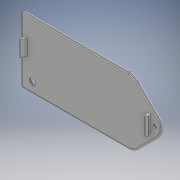
# Autodesk Inventor part: Arduino simple 4 channel ttl top
Saved by Autodesk Inventor 2017 (Build 210142000, 142)
## iProperties
Created: 2016-10-04
Part Number: Arduino simple 4 channel ttl top
Material: Generic
Document SubType Name: Modeling
Designer: andrew
Density: 1 g/cm^3
Appearance: Default
Author: andrew
Autodesk Inventor part; units mm, degrees
ref_plane "YZ Plane" through (0, 0, 0) normal (1, 0, 0) x (0, 1, 0)
ref_plane "XZ Plane" through (0, 0, 0) normal (0, 1, 0) x (-1, 0, 0)
ref_plane "XY Plane" through (0, 0, 0) normal (0, 0, 1) x (1, 0, 0)
sketch "Sketch1" plane through (0, 0, 0) normal (0, 1, 0) x (-1, 0, 0)
  line L0 (70.1002, -51.1999) -> (70.1002, -37.9894) construction
  line L1 (70.1002, -37.9894) -> (68.1002, -37.9894) construction
  line L2 (68.1002, -37.9894) -> (68.1002, -48.1999) construction
  arc A0 (67.1002, -49.1999) -> (68.1002, -48.1999) centre (67.1002, -48.1999) ccw construction
  line L3 (67.1002, -49.1999) -> (-5.9213, -49.1999) construction
  arc A1 (-7.3356, -48.6141) -> (-5.9213, -49.1999) centre (-5.9213, -47.1999) ccw construction
  line L4 (-7.3356, -48.6141) -> (-7.664, -48.2857) construction
  arc A2 (-7.664, -48.2857) -> (-9.0782, -47.6999) centre (-9.0782, -49.6999) ccw construction
  line L5 (-9.0782, -47.6999) -> (-35.9958, -47.6999) construction
  arc A3 (-42.0062, -45.2103) -> (-35.9958, -47.6999) centre (-35.9958, -39.1999) ccw construction
  line L6 (-42.0062, -45.2103) -> (-62.1562, -25.0603) construction
  arc A4 (-62.1562, -13.0395) -> (-62.1562, -25.0603) centre (-56.1458, -19.0499) ccw construction
  line L7 (-62.1562, -13.0395) -> (-42.0062, 7.1105) construction
  arc A5 (-35.9958, 9.6001) -> (-42.0062, 7.1105) centre (-35.9958, 1.1001) ccw construction
  line L8 (-35.9958, 9.6001) -> (-9.0782, 9.6001) construction
  arc A6 (-9.0782, 9.6001) -> (-7.664, 10.1859) centre (-9.0782, 11.6001) ccw construction
  line L9 (-7.664, 10.1859) -> (-7.3356, 10.5143) construction
  arc A7 (-5.9213, 11.1001) -> (-7.3356, 10.5143) centre (-5.9213, 9.1001) ccw construction
  line L10 (-5.9213, 11.1001) -> (67.1002, 11.1001) construction
  arc A8 (68.1002, 10.1001) -> (67.1002, 11.1001) centre (67.1002, 10.1001) ccw construction
  line L11 (68.1002, 10.1001) -> (68.1002, 5.7045) construction
  line L12 (68.1002, 5.7045) -> (70.1002, 5.7045) construction
  line L13 (70.1002, 5.7045) -> (70.1002, 13.1001) construction
  line L14 (70.1002, 13.1001) -> (-35.9958, 13.1001) construction
  arc A9 (-35.9958, 13.1001) -> (-44.4811, 9.5854) centre (-35.9958, 1.1001) ccw construction
  line L15 (-44.4811, 9.5854) -> (-64.6311, -10.5646) construction
  arc A10 (-64.6311, -10.5646) -> (-64.6311, -27.5352) centre (-56.1458, -19.0499) ccw construction
  line L16 (-64.6311, -27.5352) -> (-44.4811, -47.6852) construction
  arc A11 (-44.4811, -47.6852) -> (-35.9958, -51.1999) centre (-35.9958, -39.1999) ccw construction
  line L17 (-35.9958, -51.1999) -> (70.1002, -51.1999) construction
  line L18 (70.1002, -21.9894) -> (70.1002, -6.0043) construction
  line L19 (70.1002, -6.0043) -> (68.1002, -6.0043) construction
  line L20 (68.1002, -6.0043) -> (68.1002, -21.9894) construction
  line L21 (68.1002, -21.9894) -> (70.1002, -21.9894) construction
  line L22 (71.1002, -21.9894) -> (71.1002, -6.0043) construction
  line L23 (71.1002, 5.7045) -> (71.1002, 13.1001)
  arc A12 (71.1002, 13.1001) -> (70.1002, 14.1001) centre (70.1002, 13.1001) ccw
  line L24 (70.1002, 14.1001) -> (-35.9958, 14.1001)
  arc A13 (-35.9958, 14.1001) -> (-45.1882, 10.2925) centre (-35.9958, 1.1001) ccw
  line L25 (-45.1882, 10.2925) -> (-65.3382, -9.8575)
  arc A14 (-65.3382, -9.8575) -> (-65.3382, -28.2423) centre (-56.1458, -19.0499) ccw
  line L26 (-65.3382, -28.2423) -> (-45.1882, -48.3923)
  arc A15 (-45.1882, -48.3923) -> (-35.9958, -52.1999) centre (-35.9958, -39.1999) ccw
  line L27 (-35.9958, -52.1999) -> (70.1002, -52.1999)
  arc A16 (70.1002, -52.1999) -> (71.1002, -51.1999) centre (70.1002, -51.1999) ccw
  line L28 (71.1002, -51.1999) -> (71.1002, -37.9894)
  line L29 (71.1002, -37.9894) -> (70.1002, -37.9894) construction
  line L30 (70.1002, -37.9894) -> (70.1002, -51.1999) construction
  line L31 (70.1002, -51.1999) -> (-35.9958, -51.1999) construction
  arc A17 (-44.4811, -47.6852) -> (-35.9958, -51.1999) centre (-35.9958, -39.1999) ccw construction
  line L32 (-44.4811, -47.6852) -> (-64.6311, -27.5352) construction
  arc A18 (-64.6311, -10.5646) -> (-64.6311, -27.5352) centre (-56.1458, -19.0499) ccw construction
  line L33 (-64.6311, -10.5646) -> (-44.4811, 9.5854) construction
  arc A19 (-35.9958, 13.1001) -> (-44.4811, 9.5854) centre (-35.9958, 1.1001) ccw construction
  line L34 (-35.9958, 13.1001) -> (70.1002, 13.1001) construction
  line L35 (70.1002, 13.1001) -> (70.1002, 5.7045) construction
  line L36 (70.1002, 5.7045) -> (71.1002, 5.7045) construction
  line L37 (71.1002, 5.7045) -> (71.1002, 13.1001)
  line L38 (71.1002, 5.7045) -> (71.1002, -37.9894)
  arc A20 (-62.1562, -13.0395) -> (-62.1562, -25.0603) centre (-56.1458, -19.0499) ccw construction
  line L39 (-64.6458, -19.0499) -> (-76.6779, -19.0499) construction
  arc A21 (-65.3382, -9.8575) -> (-65.3382, -28.2423) centre (-56.1458, -19.0499) ccw
  circle A22 centre (-63.0458, -19.0499) radius 1.8
  point P0 (0, 0)
  point P1 (66.1, 7.6)
  point P2 (-59.329, -19.0499)
  constraints: 80 end point, 45 point on circle, 23 centre point, 1 vertical
extrude "Extrusion1" add sketch "Sketch1" along normal blind 3
sketch "Sketch2" plane through (0, 0, 0) normal (0, -1, 0) x (1, 0, 0)
  arc A0 (-71.1002, -51.1999) -> (-70.1002, -52.1999) centre (-70.1002, -51.1999) ccw projected
  line L0 (-71.1002, 13.1001) -> (-71.1002, -0.1104)
  line L1 (-70.1002, -0.1104) -> (-68.1002, -0.1104) construction
  line L2 (-68.1002, -0.1104) -> (-68.1002, 10.1001) construction
  arc A1 (-67.1002, 11.1001) -> (-68.1002, 10.1001) centre (-67.1002, 10.1001) ccw construction
  line L3 (-68.1002, -16.1104) -> (-70.1002, -16.1104) construction
  line L4 (-70.1002, -16.1104) -> (-70.1002, -32.0955) construction
  line L5 (-71.1002, -16.1104) -> (-71.1002, -32.0955) construction
  line L6 (-70.1002, -32.0955) -> (-68.1002, -32.0955) construction
  line L7 (-68.1002, -32.0955) -> (-68.1002, -16.1104) construction
  line L8 (-71.1002, -43.8043) -> (-71.1002, -0.1104)
  line L9 (-67.1002, 11.1001) -> (5.9213, 11.1001) construction
  line L10 (35.9958, 14.1001) -> (-70.1002, 14.1001)
  line L11 (35.9958, 13.1001) -> (-70.1002, 13.1001) construction
  line L12 (5.9213, -49.1999) -> (-67.1002, -49.1999) construction
  line L13 (-70.1002, -51.1999) -> (35.9958, -51.1999) construction
  line L14 (-70.1002, -52.1999) -> (35.9958, -52.1999)
  line L15 (-70.1002, 13.1001) -> (-70.1002, -0.1104) construction
  arc A2 (-70.1002, 14.1001) -> (-71.1002, 13.1001) centre (-70.1002, 13.1001) ccw
  line L16 (-68.1002, -43.8043) -> (-70.1002, -43.8043) construction
  line L17 (-68.1002, -48.1999) -> (-68.1002, -43.8043) construction
  arc A3 (-68.1002, -48.1999) -> (-67.1002, -49.1999) centre (-67.1002, -48.1999) ccw construction
  line L18 (-71.1002, -43.8043) -> (-71.1002, -51.1999)
  line L19 (-71.1002, -43.8043) -> (-71.1002, -51.1999)
  line L20 (-70.1002, -43.8043) -> (-70.1002, -51.1999) construction
  arc A4 (-71.1002, -51.1999) -> (-70.1002, -52.1999) centre (-70.1002, -51.1999) ccw
  arc A5 (5.9213, -49.1999) -> (7.3356, -48.6141) centre (5.9213, -47.1999) ccw construction
  arc A6 (9.0782, -47.6999) -> (7.664, -48.2857) centre (9.0782, -49.6999) ccw construction
  line L21 (35.9958, -47.6999) -> (9.0782, -47.6999) construction
  arc A7 (35.9958, -47.6999) -> (42.0062, -45.2103) centre (35.9958, -39.1999) ccw construction
  arc A8 (35.9958, -52.1999) -> (45.1882, -48.3923) centre (35.9958, -39.1999) ccw
  line L22 (7.664, -48.2857) -> (7.3356, -48.6141) construction
  line L23 (62.1562, -25.0603) -> (42.0062, -45.2103) construction
  line L24 (45.1882, -48.3923) -> (65.3382, -28.2423)
  arc A9 (62.1562, -25.0603) -> (62.1562, -13.0395) centre (56.1458, -19.0499) ccw construction
  arc A10 (65.3382, -28.2423) -> (65.3382, -9.8575) centre (56.1458, -19.0499) ccw
  arc A11 (7.3356, 10.5143) -> (5.9213, 11.1001) centre (5.9213, 9.1001) ccw construction
  arc A12 (7.664, 10.1859) -> (9.0782, 9.6001) centre (9.0782, 11.6001) ccw construction
  line L25 (9.0782, 9.6001) -> (35.9958, 9.6001) construction
  line L26 (7.3356, 10.5143) -> (7.664, 10.1859) construction
  line L27 (42.0062, 7.1105) -> (62.1562, -13.0395) construction
  line L28 (65.3382, -9.8575) -> (45.1882, 10.2925)
  arc A13 (42.0062, 7.1105) -> (35.9958, 9.6001) centre (35.9958, 1.1001) ccw construction
  arc A14 (44.4811, 9.5854) -> (35.9958, 13.1001) centre (35.9958, 1.1001) ccw construction
  arc A15 (45.1882, 10.2925) -> (35.9958, 14.1001) centre (35.9958, 1.1001) ccw
  line L29 (-69.6002, 12.6001) -> (35.9958, 12.6001)
  arc A16 (44.1275, 9.2318) -> (35.9958, 12.6001) centre (35.9958, 1.1001) ccw
  line L30 (44.1275, 9.2318) -> (64.2775, -10.9182)
  arc A17 (64.2775, -27.1816) -> (64.2775, -10.9182) centre (56.1458, -19.0499) ccw
  line L31 (64.2775, -27.1816) -> (44.1275, -47.3316)
  arc A18 (35.9958, -50.6999) -> (44.1275, -47.3316) centre (35.9958, -39.1999) ccw
  line L32 (35.9958, -50.6999) -> (-69.6002, -50.6999)
  line L33 (-69.6002, -50.6999) -> (-69.6002, 12.6001)
  point P0 (0, -38.0998)
  point P1 (-66.1, -45.6998)
  constraints: 68 end point, 36 point on circle, 18 centre point, 1 vertical
extrude "Extrusion2" cut sketch "Sketch2" against normal blind 1
fillet "Fillet1" radius 2 10 edges at (40.9707, 3, 13.1105) (55.2632, 3, 0.2175) (69.1458, 3, -19.0499) (55.2632, 3, -38.3173) (40.9707, 3, -51.2103) (-17.0522, 3, -52.1999) (-70.8073, 3, -51.907) (-71.1002, 3, -19.0499) (-70.8073, 3, 13.8072) (-17.0522, 3, 14.1001)
sketch "Sketch3" plane through (0, 0, 0) normal (0, -1, 0) x (1, 0, 0)
  arc A0 (65.3382, -28.2423) -> (65.3382, -9.8575) centre (56.1458, -19.0499) ccw construction
  line L0 (-70.1002, -43.8043) -> (-71.1002, -43.8043) construction
  line L1 (-70.1002, -43.8043) -> (-70.1002, -51.1999) construction
  line L2 (-70.1002, -51.1999) -> (-70.1002, -43.8043) construction
  line L3 (-68.1002, -48.1999) -> (-68.1002, -43.8043) construction
  line L4 (-68.1002, -43.8043) -> (-70.1002, -43.8043) construction
  line L5 (-70.1002, -32.0955) -> (-68.1002, -32.0955) construction
  line L6 (-71.1002, -16.1104) -> (-71.1002, -32.0955) construction
  line L7 (-70.1002, -16.1104) -> (-70.1002, -32.0955) construction
  line L8 (-68.1002, -32.0955) -> (-68.1002, -16.1104) construction
  line L9 (-68.1002, -16.1104) -> (-70.1002, -16.1104) construction
  line L10 (-71.1002, -43.8043) -> (-71.1002, -0.1104) construction
  line L11 (-70.1002, -0.1104) -> (-68.1002, -0.1104) construction
  line L12 (-68.1002, -0.1104) -> (-68.1002, 10.1001) construction
  line L13 (-70.1002, -0.1104) -> (-70.1002, 13.1001) construction
  line L14 (5.9213, -49.1999) -> (-67.1002, -49.1999) construction
  line L15 (-70.1002, -52.1999) -> (35.9958, -52.1999) construction
  line L16 (35.9958, -51.1999) -> (-70.1002, -51.1999) construction
  line L17 (-70.1002, -51.1999) -> (35.9958, -51.1999) construction
  line L18 (-67.1002, 11.1001) -> (5.9213, 11.1001) construction
  line L19 (35.9958, 13.1001) -> (-70.1002, 13.1001) construction
  line L20 (-70.1002, 13.1001) -> (35.9958, 13.1001) construction
  line L21 (35.9958, 14.1001) -> (-70.1002, 14.1001) construction
  line L22 (-71.1002, -43.8043) -> (-71.1002, -51.1999) construction
  line L23 (-71.1002, -43.8043) -> (-71.1002, -51.1999) construction
  arc A1 (-71.1002, -51.1999) -> (-70.1002, -52.1999) centre (-70.1002, -51.1999) ccw construction
  arc A2 (-68.1002, -48.1999) -> (-67.1002, -49.1999) centre (-67.1002, -48.1999) ccw construction
  arc A3 (-67.1002, 11.1001) -> (-68.1002, 10.1001) centre (-67.1002, 10.1001) ccw construction
  line L24 (-71.1002, 13.1001) -> (-71.1002, -0.1104) construction
  line L25 (-71.1002, -0.1104) -> (-70.1002, -0.1104) construction
  arc A4 (-70.1002, 14.1001) -> (-71.1002, 13.1001) centre (-70.1002, 13.1001) ccw construction
  line L26 (-70.1002, 13.1001) -> (-70.1002, -0.1104) construction
  line L27 (7.664, -48.2857) -> (7.3356, -48.6141) construction
  arc A5 (9.0782, -47.6999) -> (7.664, -48.2857) centre (9.0782, -49.6999) ccw construction
  line L28 (7.3356, 10.5143) -> (7.664, 10.1859) construction
  arc A6 (7.3356, 10.5143) -> (5.9213, 11.1001) centre (5.9213, 9.1001) ccw construction
  line L29 (35.9958, -47.6999) -> (9.0782, -47.6999) construction
  line L30 (9.0782, 9.6001) -> (35.9958, 9.6001) construction
  arc A7 (5.9213, -49.1999) -> (7.3356, -48.6141) centre (5.9213, -47.1999) ccw construction
  arc A8 (7.664, 10.1859) -> (9.0782, 9.6001) centre (9.0782, 11.6001) ccw construction
  arc A9 (64.6311, -27.5352) -> (64.6311, -10.5646) centre (56.1458, -19.0499) ccw construction
  arc A10 (35.9958, -47.6999) -> (42.0062, -45.2103) centre (35.9958, -39.1999) ccw construction
  arc A11 (35.9958, -51.1999) -> (44.4811, -47.6852) centre (35.9958, -39.1999) ccw construction
  arc A12 (35.9958, -51.1999) -> (44.4811, -47.6852) centre (35.9958, -39.1999) ccw construction
  arc A13 (35.9958, -52.1999) -> (45.1882, -48.3923) centre (35.9958, -39.1999) ccw construction
  line L31 (45.1882, -48.3923) -> (65.3382, -28.2423) construction
  line L32 (64.6311, -27.5352) -> (44.4811, -47.6852) construction
  line L33 (44.4811, -47.6852) -> (64.6311, -27.5352) construction
  arc A14 (62.1562, -25.0603) -> (62.1562, -13.0395) centre (56.1458, -19.0499) ccw construction
  arc A15 (64.6311, -27.5352) -> (64.6311, -10.5646) centre (56.1458, -19.0499) ccw construction
  arc A16 (65.3382, -28.2423) -> (65.3382, -9.8575) centre (56.1458, -19.0499) ccw construction
  line L34 (62.1562, -25.0603) -> (42.0062, -45.2103) construction
  arc A17 (42.0062, 7.1105) -> (35.9958, 9.6001) centre (35.9958, 1.1001) ccw construction
  arc A18 (44.4811, 9.5854) -> (35.9958, 13.1001) centre (35.9958, 1.1001) ccw construction
  arc A19 (44.4811, 9.5854) -> (35.9958, 13.1001) centre (35.9958, 1.1001) ccw construction
  arc A20 (45.1882, 10.2925) -> (35.9958, 14.1001) centre (35.9958, 1.1001) ccw construction
  line L35 (42.0062, 7.1105) -> (62.1562, -13.0395) construction
  line L36 (64.6311, -10.5646) -> (44.4811, 9.5854) construction
  line L37 (44.4811, 9.5854) -> (64.6311, -10.5646) construction
  line L38 (65.3382, -9.8575) -> (45.1882, 10.2925) construction
  line L39 (60.2707, -28.8292) -> (65.5374, -23.5625) construction
  circle A21 centre (63.0458, -19.0499) radius 1.6 construction
  line L40 (65.5374, -23.5625) -> (65.5374, -14.3659) construction
  arc A22 (65.3382, -28.2423) -> (65.3382, -9.8575) centre (56.1458, -19.0499) ccw construction
  line L41 (59.329, -27.8875) -> (60.2707, -28.8292) construction
  arc A23 (62.1562, -25.0603) -> (62.1562, -13.0395) centre (56.1458, -19.0499) ccw construction
  line L42 (59.329, -27.8875) -> (59.329, -10.2123) construction
  line L43 (65.5374, -14.3659) -> (59.329, -8.1575) construction
  line L44 (59.329, -8.1575) -> (59.329, -10.2123) construction
  line L45 (59.329, -19.0499) -> (80.366, -19.0499) construction
  line L46 (64.6458, -19.0499) -> (76.6779, -19.0499) construction
  line L47 (84.5257, -29.0109) -> (86.6689, -29.0109) construction
  line L48 (-67.7002, -6.1514) -> (-67.7002, -21.9095)
  line L49 (-67.7002, -21.9095) -> (-67.7002, -6.1514)
  line L50 (59.329, -27.8875) -> (58.929, -27.8875) construction
  line L51 (58.929, -27.8875) -> (58.929, -27.4875) construction
  line L52 (58.929, -27.4875) -> (56.929, -27.4875) construction
  line L53 (59.329, -10.2123) -> (58.929, -10.2123) construction
  line L54 (58.929, -10.2123) -> (58.929, -10.6123) construction
  line L55 (58.929, -27.4875) -> (58.929, -10.6123)
  line L56 (57.929, -27.4875) -> (57.929, -10.6123)
  line L57 (57.929, -27.4875) -> (58.929, -27.4875)
  line L58 (58.929, -10.6123) -> (57.929, -10.6123)
  line L59 (-66.7002, -6.1514) -> (-66.7002, -21.9095)
  line L60 (-66.7002, -21.9095) -> (-67.7002, -21.9095)
  line L61 (-66.7002, -6.1514) -> (-67.7002, -6.1514)
  line L62 (-70.1002, 14.1001) -> (35.9958, 14.1001) construction
  line L63 (-67.2002, 14.1001) -> (-67.2002, -6.0039) construction
  line L64 (-67.2002, 14.1001) -> (-47.0962, 14.1001) construction
  line L65 (-67.2002, 14.1001) -> (-67.2002, -21.9899) construction
  point P0 (-66.1, -45.6998)
  point P1 (0, -38.0998)
  dimension "d10" = 3.2
  dimension "d13" = 0.4
  dimension "d14" = 0.4
  dimension "d15" = 2
  dimension "d16" = 0.4
  dimension "d50" = 20.104
  dimension "d51" = 90
  dimension "d52" = 36.09
  constraints: 130 end point, 45 point on circle, 23 centre point, 7 perpendicular, 4 horizontal, 4 point on line, 3 parallel, 2 vertical, 1 collinear, 1 midpoint
  measures "d10" diameter of A21
  measures "d13" distance of L41.start L50.end
  measures "d14" distance of L50.end L51.end
  measures "d15" distance of L51.end L52.end
  measures "d16" distance of L53.end L54.end
  measures "d50" distance of L63.start L63.end
  measures "d51" angle of L63 L64
  measures "d52" distance of L63.start L65.end
extrude "Extrusion3" add sketch "Sketch3" along normal blind 5
sketch "Sketch7" plane through (-66.7002, 0, -21.9095) normal (0, 0, -1) x (-1, 0, 0)
  line L0 (1, 0) -> (1, -5) construction
  line L1 (1, -5) -> (1.4, -5) construction
  line L2 (1.4, -5) -> (1.9, -5) construction
  line L3 (1.9, -5) -> (1.9, -3) construction
  line L4 (1.9, -3) -> (1, -3) construction
  line L5 (1.9, -3) -> (1.9, -3.5) construction
  line L6 (1.9, -3.5) -> (0.5, -5) construction
  line L7 (0, -5) -> (1, -5) construction
  line L8 (1, -3) -> (1.9, -3)
  line L9 (1.9, -3.5) -> (1.9, -3)
  line L10 (1.9, -3.5) -> (0.5, -5)
  line L11 (0.5, -5) -> (0.5, -3)
  line L12 (0.5, -3) -> (1, -3)
  point P0 (-66.7002, 0)
  dimension "d29" = 0.4
  dimension "d30" = 0.5
  dimension "d31" = 180
  dimension "d32" = 2
  dimension "d33" = 0.5
  constraints: 22 end point, 3 collinear, 3 horizontal, 3 point on line, 1 midpoint, 1 parallel, 1 perpendicular, 1 vertical
  measures "d29" distance of L0.end L1.end
  measures "d30" distance of L1.end L2.end
  measures "d31" angle of L2 L1
  measures "d32" distance of L2.end L3.end
  measures "d33" distance of L3.end L5.end
extrude "Extrusion7" add sketch "Sketch7" against normal blind 15.758
sketch "Sketch8" plane through (-66.7002, 0, -21.9095) normal (0, 0, -1) x (-1, 0, 0)
  line L0 (1.9, -3.5) -> (1, -4.4643) projected
  line L1 (1.2, -4.25) -> (0.4365, -5.0681)
  line L2 (0.4365, -5.0681) -> (1.2, -5.0681)
  line L3 (1.2, -5.0681) -> (1.2, -4.25)
  point P0 (-66.7002, 0)
  point P1 (0.5, -5)
  constraints: 6 end point, 1 collinear, 1 horizontal, 1 perpendicular, 1 point on line
extrude "Extrusion8" cut sketch "Sketch8" against normal blind 16
sketch "Sketch9" plane through (58.929, 0, -27.4875) normal (0, 0, -1) x (-1, 0, 0)
  line L0 (125.6293, 0) -> (126.6293, 0)
  line L1 (126.6293, -3) -> (126.6293, 0)
  line L2 (128.5293, 0) -> (22.9333, 0) projected
  line L3 (126.6293, -3) -> (127.5293, -3)
  line L4 (127.5293, -3) -> (127.5293, -3.5)
  line L5 (127.5293, -3.5) -> (126.1293, -5)
  line L6 (125.6293, 0) -> (125.6293, -5) projected
  line L7 (125.6293, -5) -> (125.6293, 0)
  line L8 (-12.1673, -3.3543) -> (-13.1673, -3.3543)
  line L9 (-13.1673, -6.3543) -> (-13.1673, -3.3543)
  line L10 (-13.1673, -6.3543) -> (-14.0673, -6.3543)
  line L11 (-14.0673, -6.3543) -> (-14.0673, -6.8543)
  line L12 (-14.0673, -6.8543) -> (-12.6673, -8.3543)
  line L13 (-12.1673, -8.3543) -> (-12.1673, -3.3543)
  line L14 (-12.6673, -8.3543) -> (-12.1673, -8.3543)
  line L15 (0, -5) -> (1, -5) projected
  line L16 (-0.9, -3) -> (-0.9, -3.5)
  line L17 (0, -3) -> (0, 0)
  line L18 (0, -3) -> (-0.9, -3)
  line L19 (-0.9, -3.5) -> (0.5, -5)
  line L20 (1, 0) -> (0, 0)
  line L21 (1, -5) -> (1, 0)
  line L22 (0.5, -5) -> (1, -5)
  point P0 (58.929, 0)
  constraints: 40 end point, 2 horizontal, 2 perpendicular, 1 vertical
extrude "Extrusion9" add sketch "Sketch9" against normal blind 16.875 contours L19 L16 L18 L17 L20 L21 L15
sketch "Sketch10" plane through (58.929, 0, -27.4875) normal (0, 0, -1) x (-1, 0, 0)
  line L0 (0, -4.4643) -> (-0.9, -3.5) projected
  line L1 (-0.45, -3.9821) -> (1.0587, -5.5986)
  line L2 (1.0587, -5.5986) -> (-0.45, -5.5986)
  line L3 (-0.45, -5.5986) -> (-0.45, -3.9821)
  point P0 (58.929, 0)
  constraints: 6 end point, 1 collinear, 1 horizontal, 1 midpoint, 1 perpendicular
extrude "Extrusion10" cut sketch "Sketch10" against normal blind 20
sketch "Sketch11" plane through (0, 3, 0) normal (0, 1, 0) x (1, 0, 0)
  arc A0 (65.3382, 9.8575) -> (65.3382, 28.2423) centre (56.1458, 19.0499) ccw construction
  arc A1 (65.3382, 9.8575) -> (65.3382, 28.2423) centre (56.1458, 19.0499) ccw construction
  circle A2 centre (-50.8, 43.1) radius 1.6 construction
  line L0 (-50.8, 43.1) -> (-59.26, 43.1) construction
  line L1 (-59.26, 43.1) -> (-59.26, 41.7) construction
  circle A3 centre (-59.26, 41.7) radius 3.25
  dimension "d42" = 8.46
  dimension "d43" = 1.4
  dimension "d44" = 6.5
  constraints: 4 end point, 3 centre point, 2 point on circle, 1 coincident, 1 horizontal, 1 perpendicular
  measures "d42" distance of L0.start L0.end
  measures "d43" distance of L0.end L1.end
  measures "d44" diameter of A3
extrude "Extrusion11" cut sketch "Sketch11" against normal blind 10
chamfer "Chamfer1" distance 2 angle 45 2 edges at (-62.51, 3, -41.7) (64.8458, 3, -19.0499)
chamfer "Chamfer2" distance 2 distance2 5 1 edges at (-66.7002, 0, -14.0305) measured on face at (-66.2002, 0, -14.0305)
chamfer "Chamfer3" distance 2 distance2 5 1 edges at (57.929, 0, -19.0499) measured on face at (57.429, 0, -19.0499)
body "Solid1"
